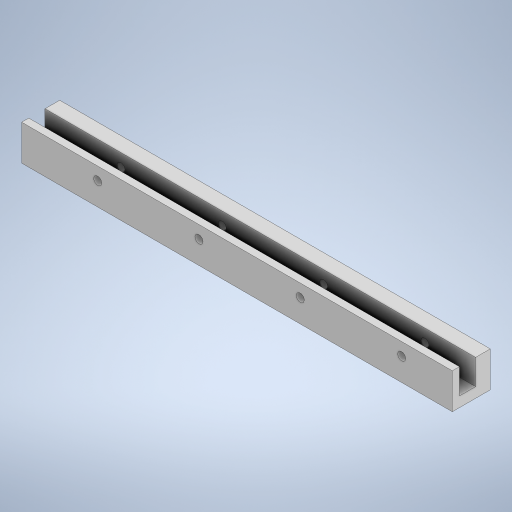
# Autodesk Inventor part: lock2
Saved by Autodesk Inventor 2023 (Build 270158000, 158)
## iProperties
Created: 2022-12-04
Part Number: lock2
Material: 一般
Document SubType Name: Modeling
Designer: RiSA
Density: 1 g/cm^3
Appearance: 既定
Author: RiSA
Autodesk Inventor part; units mm, degrees
ref_plane "YZ Plane" through (0, 0, 0) normal (1, 0, 0) x (0, 1, 0)
ref_plane "XZ Plane" through (0, 0, 0) normal (0, 1, 0) x (-1, 0, 0)
ref_plane "XY Plane" through (0, 0, 0) normal (0, 0, 1) x (1, 0, 0)
sketch "スケッチ1" plane through (0, 0, 0) normal (0, 1, 0) x (-1, 0, 0)
  line L0 (-90, -3) -> (90, -3)
  line L1 (90, -3) -> (90, 3)
  line L2 (90, 3) -> (-90, 3)
  line L3 (-90, 3) -> (-90, -3)
  line L4 (-90, -3) -> (90, 3) construction
  line L5 (90, -3) -> (-90, 3) construction
  point P0 (0, 0)
  dimension "d0" = 180
  dimension "d1" = 6
  constraints: 12 end point, 2 midpoint, 2 parallel, 1 horizontal, 1 perpendicular
  measures "d0" distance of L2.end L1.end
  measures "d1" distance of L1.end L0.end
extrude "押し出し1" add sketch "スケッチ1" along normal blind 17
sketch "スケッチ2" plane through (0, 0, 0) normal (0, -1, 0) x (1, 0, 0)
  line L0 (-90, 3) -> (90, 3) projected
  line L1 (90, 3) -> (-80, 3)
  line L2 (-80, 3) -> (-80, 9)
  line L3 (-80, 9) -> (90, 9)
  line L4 (90, 9) -> (90, 3)
  line L5 (90, 3) -> (90, -3) projected
  line L6 (90, -3) -> (-80, -3)
  line L7 (-80, -3) -> (-80, -6)
  line L8 (-80, -6) -> (90, -6)
  line L9 (90, -6) -> (90, -3)
  point P0 (0, 0)
  dimension "d4" = 170
  dimension "d5" = 6
  dimension "d6" = 170
  dimension "d7" = 3
  constraints: 16 end point, 4 parallel, 2 horizontal, 2 perpendicular
  measures "d4" distance of L2.end L3.end
  measures "d5" distance of L1.end L2.end
  measures "d6" distance of L8.end L7.end
  measures "d7" distance of L7.end L6.end
extrude "押し出し2" add sketch "スケッチ2" against normal blind 14
sketch "スケッチ3" plane through (0, 17, 0) normal (0, 1, 0) x (1, 0, 0)
  line L0 (-90, 3) -> (-90, -3) projected
  line L1 (90, -3) -> (90, 3) projected
  line L2 (-90, 3) -> (90, 3)
  line L3 (90, 3) -> (90, -3)
  line L4 (90, -3) -> (-90, -3)
  line L5 (-90, -3) -> (-90, 3)
  point P0 (0, 0)
  constraints: 8 end point, 2 parallel, 1 horizontal, 1 perpendicular
extrude "押し出し3" cut sketch "スケッチ3" against normal blind 13
sketch "スケッチ4" plane through (0, 4, 0) normal (0, 1, 0) x (1, 0, 0)
  line L0 (-90, -3) -> (-90, 3) projected
  line L1 (-80, 6) -> (-80, 3) projected
  line L2 (-90, -3) -> (-80, -3)
  line L3 (-80, -3) -> (-80, 3)
  line L4 (-80, 3) -> (-90, 3)
  line L5 (-90, 3) -> (-90, -3)
  point P0 (0, 0)
  constraints: 8 end point, 2 parallel, 1 horizontal, 1 perpendicular
extrude "押し出し4" cut sketch "スケッチ4" against normal blind 13
sketch "スケッチ5" plane through (0, 14, 0) normal (0, 1, 0) x (1, 0, 0)
  line L0 (97.0492, -3.2) -> (-97.0492, -3.2)
  line L1 (-97.0492, -3.2) -> (-97.0492, 3.2)
  line L2 (-97.0492, 3.2) -> (97.0492, 3.2)
  line L3 (97.0492, 3.2) -> (97.0492, -3.2)
  line L4 (97.0492, -3.2) -> (-97.0492, 3.2) construction
  line L5 (-97.0492, -3.2) -> (97.0492, 3.2) construction
  point P0 (0, 0)
  dimension "d14" = 6.4
  constraints: 12 end point, 2 midpoint, 2 parallel, 1 horizontal, 1 perpendicular
  measures "d14" distance of L0.end L1.end
extrude "押し出し5" cut sketch "スケッチ5" against normal blind 10
sketch "スケッチ6" plane through (-80, 0, 9) normal (0, 0, 1) x (1, 0, 0)
  line L0 (0, 14) -> (170, 14) projected
  line L1 (170, 0) -> (170, 14) projected
  point P0 (80, 0)
  point P1 (150, 9)
  point P2 (110, 9)
  point P3 (70, 9)
  point P4 (30, 9)
  dimension "d17" = 5
  dimension "d18" = 20
  dimension "d19" = 40
  dimension "d20" = 5
  dimension "d21" = 40
  dimension "d22" = 40
  measures "d17" distance from line of point (150, 9) L0
  measures "d18" distance from line of L1 point (150, 9)
  measures "d19" distance of point (150, 9) point (110, 9)
  measures "d20" distance from line of L0 point (110, 9)
  measures "d21" distance of point (110, 9) point (70, 9)
  measures "d22" distance of point (70, 9) point (30, 9)
hole "穴1" at (70, 9, 9) at (30, 9, 9) at (-10, 9, 9) at (-50, 9, 9) direction (0, 0, -1) diameter 3.2 end through all
sketch "スケッチ7" plane through (0, 0, 0) normal (0, -1, 0) x (1, 0, 0)
  line L0 (-80, -6) -> (90, -6) projected
  line L1 (90, -6) -> (90, 9) projected
  line L2 (-80, -3.2) -> (90, -3.2) projected
  point P0 (0, 0)
  point P1 (60, 0)
  point P2 (0, 0)
  point P3 (-60, 0)
  dimension "d30" = 6
  dimension "d31" = 30
  dimension "d32" = 60
  constraints: 1 coincident
  measures "d30" distance from line of L0 point (60, 0)
  measures "d31" distance from line of L1 point (60, 0)
  measures "d32" distance of point (0, 0) point (-60, 0)
hole "穴2" at (60, 0, 0) at (0, 0, 0) at (-60, 0, 0) direction (0, 1, 0) diameter 3.2 end through all
sketch "スケッチ8" plane through (90, 0, -6) normal (0, 0, -1) x (-1, 0, 0)
  line L0 (170, 0) -> (170, 14) projected
  line L1 (0, 0) -> (170, 0)
  line L2 (170, 0) -> (170, 14)
  line L3 (170, 14) -> (0, 14)
  line L4 (0, 14) -> (0, 0)
  point P0 (90, 0)
  constraints: 8 end point, 2 parallel, 1 horizontal, 1 perpendicular
extrude "押し出し6" add sketch "スケッチ8" along normal blind 3
sketch "スケッチ10" plane through (-80, 0, 9) normal (0, 0, 1) x (1, 0, 0)
  circle A0 centre (150, 9) radius 1.6 projected
  circle A1 centre (110, 9) radius 1.6 projected
  circle A2 centre (70, 9) radius 1.6 projected
  circle A3 centre (30, 9) radius 1.6 projected
  point P0 (80, 0)
  constraints: 4 coincident
hole "穴3" at (70, 9, 9) at (30, 9, 9) at (-10, 9, 9) at (-50, 9, 9) direction (0, 0, -1) diameter 3.2 end through all
sketch "スケッチ11" plane through (0, 14, 0) normal (0, 1, 0) x (1, 0, 0)
  line L0 (-80, -9) -> (90, -9) projected
  line L1 (-80, -9) -> (90, -9)
  line L2 (90, -9) -> (90, -6)
  line L3 (90, -6) -> (-80, -6)
  line L4 (-80, -6) -> (-80, -9)
  point P0 (0, 0)
  dimension "d49" = 170
  dimension "d50" = 3
  constraints: 8 end point, 2 parallel, 1 horizontal, 1 perpendicular
  measures "d49" distance of L3.end L2.end
  measures "d50" distance of L2.end L1.end
extrude "押し出し7" cut sketch "スケッチ11" against normal blind 40
